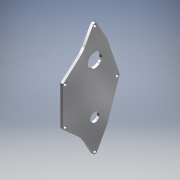
# Autodesk Inventor part: Left Plate
Saved by Autodesk Inventor 2019.4 (Build 234330000, 330)
## iProperties
Created: 2020-01-24
Part Number: Left Plate
Material: Aluminum 6061
Document SubType Name: Modeling
Designer: Mark
Mass: 166.743 g
Surface Area: 295.024 cm^2
Volume: 61.7567 cm^3
Density: 2.7 g/cm^3
Appearance: Aluminum - Flat
Author: Mark
Autodesk Inventor part; units mm, degrees
ref_plane "YZ Plane" through (0, 0, 0) normal (1, 0, 0) x (0, 1, 0)
ref_plane "XZ Plane" through (0, 0, 0) normal (0, 1, 0) x (-1, 0, 0)
ref_plane "XY Plane" through (0, 0, 0) normal (0, 0, 1) x (1, 0, 0)
sketch "Sketch7" plane through (0, 50.1691, -7.702) normal (1, 0, 0) x (0, 1, 0)
  line L0 (-25, -25) -> (25, -25) construction
  line L1 (25, -25) -> (25, 25) construction
  line L2 (25, 25) -> (-25, 25) construction
  line L3 (-25, 25) -> (-25, -25) construction
  line L4 (-25, -25) -> (25, 25) construction
  line L5 (25, -25) -> (-25, 25) construction
  line L6 (-25, -25) -> (-125, -25) construction
  line L7 (-125, -25) -> (-125, 25) construction
  line L8 (-125, 25) -> (-25, 25) construction
  line L9 (-25, 25) -> (-25, -25) construction
  circle A0 centre (0, 0) radius 14.2875
  circle A1 centre (-12.5, 60) radius 2.75
  circle A2 centre (-87.5, 60) radius 2.75
  circle A3 centre (-160, 0) radius 2.75
  circle A4 centre (60, 0) radius 2.75
  circle A5 centre (-50, -45) radius 2.75
  arc A6 (-9.3122, 63.852) -> (-12.5, 65) centre (-12.5, 60) ccw
  arc A7 (-87.5, 65) -> (-91.2516, 63.3053) centre (-87.5, 60) ccw
  arc A8 (61.8932, -4.6277) -> (62.4135, 4.3789) centre (60, 0) ccw
  arc A9 (-51.8932, -49.6277) -> (-48.1068, -49.6277) centre (-50, -45) ccw
  arc A10 (-163.1878, 3.852) -> (-161.8932, -4.6277) centre (-160, 0) ccw
  line L10 (-12.5, 65) -> (-87.5, 65)
  circle A11 centre (-100, 0) radius 9.5
  line L11 (-163.1878, 3.852) -> (-90.6878, 63.852)
  line L12 (-9.3122, 63.852) -> (63.1878, 3.852)
  line L13 (-161.8932, -4.6277) -> (-51.8932, -49.6277)
  line L14 (-48.1068, -49.6277) -> (61.8932, -4.6277)
  circle A12 centre (0, 0) radius 25.4 construction
  circle A13 centre (17.9605, 17.9605) radius 2.75
  circle A14 centre (-17.9605, -17.9605) radius 2.75
  dimension "d110" = 50
  dimension "d107" = 100
  dimension "d108" = 50
  dimension "d106" = 28.575
  dimension "d104" = 5.5
  dimension "d101" = 5.5
  dimension "d98" = 5.5
  dimension "d95" = 5.5
  dimension "d92" = 5.5
  dimension "d94" = 75
  dimension "d93" = 20
  dimension "d100" = 35
  dimension "d97" = 35
  dimension "d96" = 25
  dimension "d103" = 35
  dimension "d102" = 37.5
  dimension "d99" = 25
  dimension "d105" = 37.5
  dimension "d91" = 10
  dimension "d90" = 10
  dimension "d89" = 10
  dimension "d88" = 10
  dimension "d87" = 10
  dimension "d109" = 50
  dimension "d86" = 75
  dimension "d83" = 19
  dimension "d85" = 25
  dimension "d84" = 25
  dimension "d114" = 50.8
  dimension "d115" = 5.5
  dimension "d116" = 5.5
  constraints: 30 end point, 15 centre point, 14 point on circle, 10 tangent, 7 coincident, 4 parallel, 2 horizontal, 2 midpoint, 2 perpendicular, 2 point on line
  measures "d110" distance of L1.end L0.end
  measures "d107" distance of L7.end L8.end
  measures "d108" distance of L6.end L7.end
  measures "d106" diameter of A0
  measures "d104" diameter of A1
  measures "d101" diameter of A2
  measures "d98" diameter of A3
  measures "d95" diameter of A4
  measures "d92" diameter of A5
  measures "d94" distance from line of L1 A5.centre
  measures "d93" distance from line of L6 A5.centre
  measures "d100" distance from line of L7 A3.centre
  measures "d97" distance from line of L1 A4.centre
  measures "d96" distance from line of L0 A4.centre
  measures "d103" distance from line of L8 A2.centre
  measures "d102" distance from line of L7 A2.centre
  measures "d99" distance from line of L8 A3.centre
  measures "d105" distance from line of L1 A1.centre
  measures "d91" diameter of A6
  measures "d90" diameter of A7
  measures "d89" diameter of A8
  measures "d88" diameter of A9
  measures "d87" diameter of A10
  measures "d109" distance of L1.end L2.end
  measures "d86" distance of L10.start L10.end
  measures "d83" diameter of A11
  measures "d85" distance from line of L6 A11.centre
  measures "d84" distance from line of L7 A11.centre
  measures "d114" diameter of A12
  measures "d115" diameter of A13
  measures "d116" diameter of A14
extrude "Extrusion7" add sketch "Sketch7" along normal blind 5
body "Solid4"
